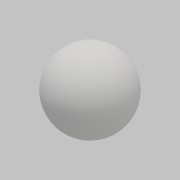
# Autodesk Inventor part: 彈珠檯球
Saved by Autodesk Inventor 2018 (Build 220112000, 112)
## iProperties
Created: 2020-12-11
Part Number: 彈珠檯球
Material: 一般
Document SubType Name: Modeling
Designer: 王鼎鈞
Density: 1 g/cm^3
Appearance: 預設
Author: 王鼎鈞
Autodesk Inventor part; units mm, degrees
ref_plane "YZ Plane" through (0, 0, 0) normal (1, 0, 0) x (0, 1, 0)
ref_plane "XZ Plane" through (0, 0, 0) normal (0, 1, 0) x (-1, 0, 0)
ref_plane "XY Plane" through (0, 0, 0) normal (0, 0, 1) x (1, 0, 0)
sketch "草圖1" plane through (0, 0, 0) normal (1, 0, 0) x (0, 1, 0)
  arc A0 (-2.5, 0) -> (2.5, 0) centre (0, 0) ccw
  line L0 (-3.5, 0) -> (3.5, 0) projected
  line L1 (0, -3) -> (0, 0.5) projected
  dimension "d0" = 5
  constraints: 2 point on circle, 2 point on line, 1 centre point, 1 coincident
  measures "d0" diameter of A0
revolve "迴轉1" add sketch "草圖1" angle 360 about axis through (0, -10, 0) along (0, 1, 0)
